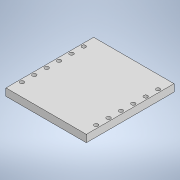
# Autodesk Inventor part: Драйвер моторов DRV8833
Saved by Autodesk Inventor 2020 (Build 240168000, 168)
## iProperties
Created: 2021-08-09
Part Number: Драйвер моторов DRV8833
Material: Типовые
Document SubType Name: Modeling
Designer: Антон
Density: 1 g/cm^3
Appearance: По умолчанию
Author: Антон
Autodesk Inventor part; units mm, degrees
ref_plane "YZ Plane" through (0, 0, 0) normal (1, 0, 0) x (0, 1, 0)
ref_plane "XZ Plane" through (0, 0, 0) normal (0, 1, 0) x (-1, 0, 0)
ref_plane "XY Plane" through (0, 0, 0) normal (0, 0, 1) x (1, 0, 0)
sketch "Эскиз1" plane through (0, 0, 0) normal (0, 1, 0) x (-1, 0, 0)
  line L0 (0, 0) -> (16.5, 0)
  line L1 (16.5, 0) -> (16.5, -18)
  line L2 (16.5, -18) -> (0, -18)
  line L3 (0, -18) -> (0, 0)
  dimension "d0" = 16.5
  dimension "d1" = 18
  constraints: 8 end point, 2 parallel, 1 horizontal, 1 perpendicular
  measures "d0" distance of L1.end L2.end
  measures "d1" distance of L0.end L1.end
extrude "Выдавливание1" add sketch "Эскиз1" along normal blind 1.5
sketch "Эскиз2" plane through (0, 1.5, 0) normal (0, 1, 0) x (1, 0, 0)
  line L0 (-16.5, 18) -> (-16.5, 0) projected
  line L1 (-16.5, 0) -> (0, 0) construction
  line L2 (-8.25, 0) -> (-8.25, 18) construction
  line L3 (0, 18) -> (-16.5, 18) construction
  line L4 (-15.87, 2.65) -> (-15.87, 0) construction
  line L5 (-15.87, 15.35) -> (-15.87, 18) construction
  line L6 (-15.87, 2.65) -> (-16.5, 2.65) construction
  point P0 (-15.87, 12.81)
  point P1 (-15.87, 10.27)
  point P2 (-15.87, 7.73)
  point P3 (-15.87, 5.19)
  point P4 (-0.63, 15.35)
  point P5 (-0.63, 12.81)
  point P6 (-0.63, 10.27)
  point P7 (-0.63, 7.73)
  point P8 (-0.63, 5.19)
  point P9 (-0.63, 2.65)
  dimension "d6" = 2.54
  dimension "d11" = 15.24
  constraints: 8 end point, 6 symmetric about line, 3 point on line, 2 midpoint, 2 perpendicular, 2 vertical, 1 collinear, 5 other
  measures "d6" distance of L5.start point (-15.87, 12.81)
  measures "d11" distance of point (-0.63, 2.65) L4.start
hole "Отверстие1" at (-15.87, 1.5, -15.35) at (-15.87, 1.5, -12.81) at (-15.87, 1.5, -10.27) at (-15.87, 1.5, -7.73) at (-15.87, 1.5, -5.19) at (-15.87, 1.5, -2.65) at (-0.63, 1.5, -2.65) at (-0.63, 1.5, -5.19) at (-0.63, 1.5, -7.73) at (-0.63, 1.5, -10.27) at (-0.63, 1.5, -12.81) at (-0.63, 1.5, -15.35) direction (0, -1, 0) diameter 0.8 end through all
